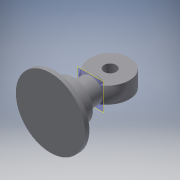
# Autodesk Inventor part: cast2
Saved by Autodesk Inventor 2016 (Build 200138000, 138)
## iProperties
Created: 2016-11-29
Part Number: cast2
Material: Generic
Document SubType Name: Modeling
Designer: Juraj
Density: 1 g/cm^3
Appearance: Default
Author: Juraj
Autodesk Inventor part; units mm, degrees
ref_plane "YZ Plane" through (0, 0, 0) normal (1, 0, 0) x (0, 1, 0)
ref_plane "XZ Plane" through (0, 0, 0) normal (0, 1, 0) x (-1, 0, 0)
ref_plane "XY Plane" through (0, 0, 0) normal (0, 0, 1) x (1, 0, 0)
sketch "Sketch1" plane through (0, 0, 0) normal (0, 0, 1) x (1, 0, 0)
  circle A0 centre (0, 0) radius 8
  dimension "d0" = 16
  constraints: 1 centre point, 1 coincident
  measures "d0" diameter of A0
extrude "Extrusion1" add sketch "Sketch1" along normal blind 1
sketch "Sketch2" plane through (0, 0, 0) normal (0, 0, -1) x (-1, 0, 0)
  circle A0 centre (0, 0) radius 4.5
  dimension "d3" = 9
  constraints: 1 centre point, 1 coincident
  measures "d3" diameter of A0
extrude "Extrusion2" add sketch "Sketch2" along normal blind 4.3
sketch "Sketch3" plane through (0, 0, -4.3) normal (0, 0, -1) x (-1, 0, 0)
  circle A0 centre (0, 0) radius 8 projected
  circle A1 centre (0, 0) radius 2.8
  dimension "d6" = 5.6
  constraints: 1 centre point, 1 coincident
  measures "d6" diameter of A1
extrude "Extrusion3" add sketch "Sketch3" along normal blind 5 contours A1
ref_plane "Work Plane1" through (0, 0, -8.3) normal (0, 0, -1) x (-1, 0, 0)
sketch "Sketch4" plane through (0, 0, -8.3) normal (0, 0, -1) x (-1, 0, 0)
  line L0 (-4.5, -1.9) -> (4.5, -1.9)
  line L1 (4.5, -1.9) -> (4.5, 1.9)
  line L2 (4.5, 1.9) -> (-4.5, 1.9)
  line L3 (-4.5, 1.9) -> (-4.5, -1.9)
  circle A0 centre (0, 0) radius 2.8 projected
  circle A1 centre (0, 0) radius 8 projected
  dimension "d10" = 9
  dimension "d11" = 3.8
  dimension "d12" = 1.9
  dimension "d13" = 4.5
  constraints: 8 end point, 2 parallel, 1 horizontal, 1 perpendicular
  measures "d10" distance of L2.end L1.end
  measures "d11" distance of L0.end L1.end
  measures "d12" distance from line of L2 A0.centre
  measures "d13" distance from line of A1.centre L1
extrude "Extrusion4" add sketch "Sketch4" along normal blind 9 contours L3 L2 A0 L0 | A0 L2 L0 | A0 L2 L1 L0
fillet "Fillet1" radius 4.4 4 edges at (-4.5, 0, -8.3) (4.5, 0, -8.3) (4.5, 0, -17.3) (-4.5, 0, -17.3)
sketch "Sketch5" plane through (-2.0567, -1.9, -9.3) normal (0, -1, 0) x (1, 0, 0)
  arc A0 (-2.4433, -3.6) -> (1.9567, -8) centre (1.9567, -3.6) ccw projected
  circle A1 centre (1.9567, -3.6) radius 1.4
  point P0 (2.0567, 9.3)
  dimension "d18" = 2.8
  dimension "d19" = 4.4
  constraints: 1 centre point
  measures "d18" diameter of A1
  measures "d19" distance of A0.end A1.centre
extrude "Extrusion5" cut sketch "Sketch5" against normal blind 9
sketch "Sketch6" plane through (0, 0, 1) normal (0, 0, 1) x (1, 0, 0)
  circle A0 centre (0, 0) radius 1.5
  dimension "d22" = 3
  constraints: 1 centre point, 1 coincident
  measures "d22" diameter of A0
extrude "Extrusion6" add sketch "Sketch6" along normal blind 15
fillet "Fillet2" radius 0.5 1 edges at (-1.5, 0, 16)
fillet "Fillet3" radius 0.5 4 edges at (-8, 0, 0) (4.5, 0, -4.3) (0, 2.8, -9.3) (0, -2.8, -9.3)
fillet "Fillet4" radius 0.5 14 edges at (0, 1.9, -17.3) (3.2113, 1.9, -16.0113) (4.5, 1.9, -12.7538) (3.6737, 1.9, -9.9013) (-4.5, 1.9, -12.7538) (-3.6737, 1.9, -9.9013) (-3.2113, 1.9, -16.0113) (-4.5, -1.9, -12.7538) (-3.6737, -1.9, -9.9013) (0, -1.9, -17.3) (3.2113, -1.9, -16.0113) (4.5, -1.9, -12.7538) (3.6737, -1.9, -9.9013) (-3.2113, -1.9, -16.0113)
equation "\"d12\" = 0.5 * d11"
equation "\"d13\" = 0.5 * d10"
body "Solid1"
